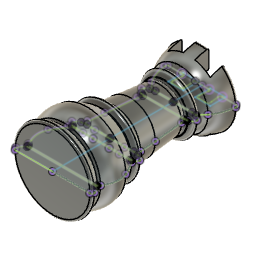
Rook v1 (Autodesk Fusion 360 design; units mm, degrees)
Autodesk Fusion 360 part; units mm, degrees
sketch "Sketch1" plane through (0, 0, 0) normal (0, 0, 1) x (1, 0, 0)
  spline S0 degree 3 poles (56.456539, 22.484084) (57.156363, 22.57219) (57.847984, 22.484877) (58.537222, 22.508691) knots 0 0 0 0 1 1 1 1
  spline S1 degree 3 poles (58.537222, 22.508691) (58.763177, 22.516363) (58.702853, 22.354174) (58.697031, 22.252309) knots 0 0 0 0 1 1 1 1
  spline S2 degree 3 poles (58.697031, 22.252309) (58.67322, 21.863107) (58.623744, 21.475229) (58.598079, 21.086026) knots 0 0 0 0 1 1 1 1
  spline S3 degree 3 poles (58.598079, 21.086026) (58.582996, 20.853723) (58.580618, 20.671953) (58.947593, 20.719578) knots 0 0 0 0 1 1 1 1
  spline S4 degree 3 poles (58.947593, 20.719578) (59.209795, 20.753444) (59.503749, 20.742332) (59.773887, 20.712434) knots 0 0 0 0 1 1 1 1
  spline S5 degree 3 poles (59.773887, 20.712434) (60.200662, 20.665073) (60.237966, 20.861395) (60.18505, 21.195829) knots 0 0 0 0 1 1 1 1
  spline S6 degree 3 poles (60.18505, 21.195829) (60.133454, 21.521267) (60.12102, 21.853318) (60.065988, 22.177961) knots 0 0 0 0 1 1 1 1
  spline S7 degree 3 poles (60.065988, 22.177961) (60.023654, 22.427199) (60.126313, 22.516099) (60.35253, 22.515834) knots 0 0 0 0 1 1 1 1
  spline S8 degree 3 poles (60.35253, 22.515834) (60.976418, 22.515041) (61.600835, 22.513981) (62.224194, 22.510277) knots 0 0 0 0 1 1 1 1
  spline S9 degree 3 poles (62.224194, 22.510277) (62.435595, 22.509219) (62.55651, 22.462917) (62.509149, 22.18775) knots 0 0 0 0 1 1 1 1
  spline S10 degree 3 poles (62.509149, 22.18775) (62.338229, 21.195827) (62.099311, 20.209461) (61.466161, 19.424177) knots 0 0 0 0 1 1 1 1
  spline S11 degree 3 poles (61.466161, 19.424177) (61.153689, 19.037092) (60.831954, 18.580155) (60.102764, 18.618255) knots 0 0 0 0 1 1 1 1
  spline S12 degree 3 poles (60.102764, 18.618255) (58.379266, 18.708212) (56.648097, 18.640746) (54.920106, 18.632805) knots 0 0 0 0 1 1 1 1
  spline S13 degree 3 poles (54.920106, 18.632805) (54.658696, 18.631747) (54.426657, 18.681752) (54.236156, 18.877545) knots 0 0 0 0 1 1 1 1
  spline S14 degree 3 poles (54.236156, 18.877545) (53.326518, 19.815493) (52.892868, 20.96405) (52.749728, 22.23987) knots 0 0 0 0 1 1 1 1
  spline S15 degree 3 poles (52.749728, 22.23987) (52.735707, 22.362372) (52.676703, 22.530647) (52.922234, 22.526414) knots 0 0 0 0 1 1 1 1
  spline S16 degree 3 poles (52.922234, 22.526414) (53.561734, 22.515302) (54.201759, 22.517153) (54.841521, 22.515566) knots 0 0 0 0 1 1 1 1
  spline S17 degree 3 poles (54.841521, 22.515566) (55.083084, 22.514773) (55.194475, 22.428253) (55.153728, 22.158379) knots 0 0 0 0 1 1 1 1
  spline S18 degree 3 poles (55.153728, 22.158379) (55.095786, 21.773674) (55.075939, 21.38315) (55.035724, 20.9958) knots 0 0 0 0 1 1 1 1
  spline S19 degree 3 poles (55.035724, 20.9958) (55.019054, 20.840491) (55.031489, 20.687296) (55.22834, 20.70661) knots 0 0 0 0 1 1 1 1
  spline S20 degree 3 poles (55.22834, 20.70661) (55.642942, 20.747885) (56.060984, 20.639936) (56.475587, 20.749738) knots 0 0 0 0 1 1 1 1
  spline S21 degree 3 poles (56.475587, 20.749738) (56.580627, 20.777784) (56.661323, 20.764026) (56.646244, 20.908487) knots 0 0 0 0 1 1 1 1
  spline S22 degree 3 poles (56.646244, 20.908487) (56.591209, 21.428132) (56.617402, 21.957033) (56.456539, 22.484084) knots 0 0 0 0 1 1 1 1
  line L0 (62.280812, 3.156799) -> (52.878314, 3.156799)
  spline S23 degree 3 poles (52.878314, 3.156799) (52.587008, 3.053612) (52.435136, 2.800139) (52.282472, 2.325741) knots 0 0 0 0 1 1 1 1
  spline S24 degree 3 poles (52.282472, 2.325741) (52.173992, 1.988399) (52.268184, 1.946856) (52.556579, 1.947652) knots 0 0 0 0 1 1 1 1
  spline S25 degree 3 poles (52.556579, 1.947652) (54.118415, 1.953473) (55.68025, 1.953207) (57.241819, 1.952149) knots 0 0 0 0 1 1 1 1
  spline S26 degree 3 poles (57.241819, 1.952149) (59.060034, 1.950825) (60.877458, 1.951354) (62.694882, 1.939185) knots 0 0 0 0 1 1 1 1
  spline S27 degree 3 poles (62.694882, 1.939185) (62.988569, 1.93707) (63.017936, 2.059043) (62.963434, 2.299814) knots 0 0 0 0 1 1 1 1
  spline S28 degree 3 poles (62.963434, 2.299814) (62.85046, 2.797495) (62.650169, 3.059434) (62.280812, 3.156799) knots 0 0 0 0 1 1 1 1
  line L1 (54.363684, 17.329206) -> (60.721888, 17.329206)
  spline S29 degree 3 poles (60.721888, 17.329206) (60.74861, 17.332117) (60.774803, 17.334499) (60.801263, 17.33873) knots 0 0 0 0 1 1 1 1
  spline S30 degree 3 poles (60.801263, 17.33873) (61.148662, 17.392441) (61.432293, 17.710469) (61.383875, 17.990927) knots 0 0 0 0 1 1 1 1
  spline S31 degree 3 poles (61.383875, 17.990927) (61.323284, 18.342823) (61.112412, 18.510303) (60.744375, 18.508717) knots 0 0 0 0 1 1 1 1
  spline S32 degree 3 poles (60.744375, 18.508717) (58.68433, 18.498135) (56.624282, 18.493634) (54.564503, 18.493634) knots 0 0 0 0 1 1 1 1
  spline S33 degree 3 poles (54.564503, 18.493634) (54.29357, 18.493634) (54.06841, 18.427488) (53.955432, 18.169255) knots 0 0 0 0 1 1 1 1
  spline S34 degree 3 poles (53.955432, 18.169255) (53.80012, 17.81419) (54.004379, 17.450121) (54.363684, 17.329206) knots 0 0 0 0 1 1 1 1
  spline S35 degree 3 poles (61.03277, 12.609569) (60.880635, 13.946245) (60.75972, 15.284769) (60.63325, 16.623298) knots 0 0 0 0 1 1 1 1
  spline S36 degree 3 poles (60.63325, 16.623298) (60.597004, 17.008001) (60.577953, 17.137119) (60.39195, 17.178925) knots 0 0 0 0 1 1 1 1
  line L2 (60.39195, 17.178925) -> (54.82882, 17.178925)
  spline S37 degree 3 poles (54.82882, 17.178925) (54.745742, 17.150087) (54.684356, 17.080235) (54.671393, 16.909315) knots 0 0 0 0 1 1 1 1
  spline S38 degree 3 poles (54.671393, 16.909315) (54.606834, 16.020844) (54.513965, 15.134226) (54.427977, 14.247607) knots 0 0 0 0 1 1 1 1
  spline S39 degree 3 poles (54.427977, 14.247607) (54.289601, 12.822561) (54.14699, 11.398044) (54.003584, 9.94072) knots 0 0 0 0 1 1 1 1
  spline S40 degree 3 poles (54.003584, 9.94072) (54.767701, 9.94072) (55.54531, 9.941778) (56.323452, 9.94072) knots 0 0 0 0 1 1 1 1
  spline S41 degree 3 poles (56.323452, 9.94072) (57.814644, 9.939133) (59.30557, 9.945746) (60.796233, 9.927756) knots 0 0 0 0 1 1 1 1
  spline S42 degree 3 poles (60.796233, 9.927756) (61.150774, 9.923259) (61.249992, 10.040734) (61.223537, 10.385222) knots 0 0 0 0 1 1 1 1
  spline S43 degree 3 poles (61.223537, 10.385222) (61.167181, 11.127639) (61.116643, 11.875348) (61.03277, 12.609569) knots 0 0 0 0 1 1 1 1
  line L3 (53.457485, 8.771787) -> (53.993002, 8.771787)
  spline S44 degree 3 poles (53.993002, 8.771787) (53.999087, 8.771787) (54.004908, 8.771787) (54.010992, 8.771787) knots 0 0 0 0 1 1 1 1
  line L4 (54.010992, 8.771787) -> (61.651365, 8.771787)
  spline S45 degree 3 poles (61.651365, 8.771787) (62.032894, 8.81465) (62.241122, 8.99192) (62.229479, 9.265765) knots 0 0 0 0 1 1 1 1
  spline S46 degree 3 poles (62.229479, 9.265765) (62.215191, 9.602845) (61.949284, 9.787257) (61.473566, 9.788848) knots 0 0 0 0 1 1 1 1
  spline S47 degree 3 poles (61.473566, 9.788848) (60.849944, 9.791492) (60.22579, 9.792021) (59.602168, 9.793612) knots 0 0 0 0 1 1 1 1
  spline S48 degree 3 poles (59.602168, 9.793612) (58.091929, 9.796256) (56.581951, 9.800491) (55.071441, 9.80102) knots 0 0 0 0 1 1 1 1
  spline S49 degree 3 poles (55.071441, 9.80102) (54.615562, 9.801815) (54.160216, 9.793612) (53.704341, 9.788319) knots 0 0 0 0 1 1 1 1
  spline S50 degree 3 poles (53.704341, 9.788319) (53.337099, 9.783821) (53.15586, 9.54596) (53.153478, 9.229785) knots 0 0 0 0 1 1 1 1
  spline S51 degree 3 poles (53.153478, 9.229785) (53.151625, 8.997742) (53.253755, 8.832111) (53.457485, 8.771787) knots 0 0 0 0 1 1 1 1
  spline S52 degree 3 poles (62.913429, 6.665177) (62.658635, 7.290651) (62.269169, 7.834901) (61.951403, 8.421744) knots 0 0 0 0 1 1 1 1
  spline S53 degree 3 poles (61.951403, 8.421744) (61.854566, 8.600601) (61.692375, 8.613039) (61.520397, 8.612773) knots 0 0 0 0 1 1 1 1
  spline S54 degree 3 poles (61.520397, 8.612773) (61.033299, 8.612773) (60.545937, 8.612506) (60.058839, 8.612506) knots 0 0 0 0 1 1 1 1
  spline S55 degree 3 poles (60.058839, 8.612506) (59.59476, 8.61224) (59.130944, 8.612506) (58.667132, 8.612506) knots 0 0 0 0 1 1 1 1
  spline S56 degree 3 poles (58.667132, 8.612506) (58.667132, 8.61568) (58.667132, 8.618328) (58.667132, 8.621501) knots 0 0 0 0 1 1 1 1
  line L5 (58.667132, 8.621501) -> (53.760168, 8.621501)
  spline S57 degree 3 poles (53.760168, 8.621501) (53.698786, 8.6088) (53.644017, 8.580225) (53.600625, 8.516727) knots 0 0 0 0 1 1 1 1
  spline S58 degree 3 poles (53.600625, 8.516727) (53.178085, 7.898661) (52.733587, 7.289327) (52.377722, 6.633158) knots 0 0 0 0 1 1 1 1
  spline S59 degree 3 poles (52.377722, 6.633158) (51.942482, 5.830146) (52.09938, 4.976601) (52.392272, 4.166448) knots 0 0 0 0 1 1 1 1
  spline S60 degree 3 poles (52.392272, 4.166448) (52.594679, 3.606324) (52.723002, 3.404713) (53.074369, 3.344651) knots 0 0 0 0 1 1 1 1
  line L6 (53.074369, 3.344651) -> (62.303037, 3.344651)
  spline S61 degree 3 poles (62.303037, 3.344651) (62.392466, 3.378782) (62.473694, 3.443075) (62.538782, 3.560021) knots 0 0 0 0 1 1 1 1
  spline S62 degree 3 poles (62.538782, 3.560021) (63.085939, 4.542951) (63.367188, 5.551546) (62.913429, 6.665177) knots 0 0 0 0 1 1 1 1
  line L7 (57.560832, 22.519067) -> (57.560832, 1.951933)
  constraint perpendicular L0 L7
revolve "Revolve1" add sketch "Sketch1" angle 360 about axis through (57.560832, 22.519067, 0) along (0, -1, 0) contours S0 S1 S2 S3 S4 S5 S6 S7 S8 S9 S10 S11 S12 L7 | L0 S26 S27 S28 L7 | L1 S29 S30 S31 S32 L7 | S35 S36 L2 S41 S42 S43 L7 | L4 S45 S46 S47 S48 L7 | S52 S53 S54 S55 S56 L5 L6 S61 S62 L7 picked at (58.843066, 19.331093) picked at (60.845509, 2.349306) picked at (59.675698, 18.111637) picked at (58.718145, 13.243028) picked at (59.604789, 9.112395) picked at (59.974236, 5.100603) makes body 1 at (58.916375, 8.771787, 0.750935) makes body 2 at (60.984842, 20.949003, 3.177016) makes body 3 at (54.215916, 4.393756, -4.194392) makes body 4 at (60.885542, 13.946793, -0.165929) makes body 5 at (55.173184, 18.504928, 0) makes body 6 at (53.710141, 1.945857, 0)
sketch "Sketch2" plane through (0, 0, 0) normal (0, 0, 1) x (1, 0, 0)
  spline S0 degree 3 poles (58.537222, 22.508691) (58.374743, 22.503077) (58.212157, 22.503642) (57.88746, 22.509584) (57.725237, 22.514953) (57.562009, 22.519037) (57.561421, 22.519052) (57.560832, 22.519067) knots -0.09770796 -0.09770796 -0.09770796 -0.09770796 -0.04880692 -0.04880692 0 0 0.0001766 0.0001766 0.0001766 0.0001766
  spline S1 degree 3 poles (57.560832, 22.519067) (57.560244, 22.519052) (57.559655, 22.519037) (57.396428, 22.514953) (57.234205, 22.509584) (56.909507, 22.503642) (56.746921, 22.503077) (56.584443, 22.508691) knots -0.09762764 -0.09762764 -0.09762764 -0.09762764 -0.0974515 -0.0974515 -0.04877269 -0.04877269 0 0 0 0
  spline S2 degree 3 poles (54.769134, 22.515834) (54.457108, 22.515438) (54.145089, 22.514974) (53.521297, 22.513321) (53.209294, 22.51213) (52.89747, 22.510277) knots -0.18715063 -0.18715063 -0.18715063 -0.18715063 -0.09354867 -0.09354867 0 0 0 0
  spline S3 degree 3 poles (52.89747, 22.510277) (52.827114, 22.509925) (52.766785, 22.504562) (52.69966, 22.480309) (52.680993, 22.470735) (52.648886, 22.44481) (52.636343, 22.429528) (52.615182, 22.390035) (52.607851, 22.364537) (52.599958, 22.295101) (52.602344, 22.246846) (52.612515, 22.18775) knots -0.0820162 -0.0820162 -0.0820162 -0.0820162 -0.0542049 -0.0542049 -0.04266662 -0.04266662 -0.03149039 -0.03149039 -0.01798963 -0.01798963 0 0 0 0
  spline S4 degree 3 poles (52.612515, 22.18775) (52.704342, 21.654838) (52.818349, 21.108717) (53.164161, 20.172799) (53.370971, 19.777077) (53.655503, 19.424177) knots -0.29910345 -0.29910345 -0.29910345 -0.29910345 -0.13599545 -0.13599545 0 0 0 0
  spline S5 degree 3 poles (53.655503, 19.424177) (53.799947, 19.245243) (53.946207, 19.051614) (54.245815, 18.807301) (54.366194, 18.73571) (54.648401, 18.634905) (54.817556, 18.607735) (55.018901, 18.618255) knots -0.21041698 -0.21041698 -0.21041698 -0.21041698 -0.11657514 -0.11657514 -0.06048604 -0.06048604 0 0 0 0
  spline S6 degree 3 poles (55.018901, 18.618255) (55.441953, 18.640336) (55.865388, 18.652927) (56.711898, 18.665556) (57.13505, 18.665613) (57.558935, 18.662608) (57.559884, 18.662601) (57.560832, 18.662594) knots -0.25395917 -0.25395917 -0.25395917 -0.25395917 -0.12688391 -0.12688391 0 0 0.00028462 0.00028462 0.00028462 0.00028462
  spline S7 degree 3 poles (57.560832, 18.662594) (57.561781, 18.662601) (57.56273, 18.662608) (57.986614, 18.665613) (58.409767, 18.665556) (59.256277, 18.652927) (59.679711, 18.640336) (60.102764, 18.618255) knots -0.25427015 -0.25427015 -0.25427015 -0.25427015 -0.2539855 -0.2539855 -0.12708844 -0.12708844 0 0 0 0
  spline S8 degree 3 poles (60.102764, 18.618255) (60.264394, 18.60981) (60.424712, 18.624709) (60.711268, 18.715367) (60.829821, 18.778654) (61.15132, 19.019589) (61.309781, 19.230456) (61.466161, 19.424177) knots -0.16022181 -0.16022181 -0.16022181 -0.16022181 -0.1140258 -0.1140258 -0.07468907 -0.07468907 0 0 0 0
  spline S9 degree 3 poles (61.466161, 19.424177) (61.780203, 19.813677) (61.999008, 20.254625) (62.322223, 21.200122) (62.424919, 21.698927) (62.509149, 22.18775) knots -0.29831003 -0.29831003 -0.29831003 -0.29831003 -0.14880799 -0.14880799 0 0 0 0
  spline S10 degree 3 poles (62.509149, 22.18775) (62.521923, 22.261968) (62.522459, 22.319552) (62.507484, 22.384982) (62.499873, 22.405049) (62.477163, 22.439951) (62.463302, 22.453882) (62.425936, 22.479352) (62.401518, 22.489107) (62.331844, 22.506403) (62.281346, 22.509991) (62.224194, 22.510277) knots -0.06670843 -0.06670843 -0.06670843 -0.06670843 -0.04653663 -0.04653663 -0.03707383 -0.03707383 -0.0281827 -0.0281827 -0.0171458 -0.0171458 0 0 0 0
  spline S11 degree 3 poles (62.224194, 22.510277) (61.912371, 22.51213) (61.600368, 22.513321) (60.976576, 22.514974) (60.664556, 22.515438) (60.35253, 22.515834) knots -0.1871624 -0.1871624 -0.1871624 -0.1871624 -0.09360785 -0.09360785 0 0 0 0
  spline S12 degree 3 poles (61.383875, 17.990927) (61.371233, 18.064349) (61.350691, 18.137626) (61.289893, 18.262797) (61.253212, 18.315101) (61.156565, 18.405554) (61.099173, 18.439486) (60.943653, 18.497621) (60.84244, 18.509139) (60.744375, 18.508717) knots -0.09136626 -0.09136626 -0.09136626 -0.09136626 -0.06904077 -0.06904077 -0.04970491 -0.04970491 -0.02941973 -0.02941973 0 0 0 0
  spline S13 degree 3 poles (60.744375, 18.508717) (60.213782, 18.505991) (59.683186, 18.503669) (58.623067, 18.499782) (58.093541, 18.498215) (57.562954, 18.496993) (57.561893, 18.496991) (57.560832, 18.496988) knots -0.31803786 -0.31803786 -0.31803786 -0.31803786 -0.15885803 -0.15885803 0 0 0.00031833 0.00031833 0.00031833 0.00031833
  spline S14 degree 3 poles (57.560832, 18.496988) (57.559771, 18.496991) (57.55871, 18.496993) (57.028124, 18.498215) (56.498597, 18.499782) (55.438478, 18.503669) (54.907882, 18.505991) (54.37729, 18.508717) knots -0.31835618 -0.31835618 -0.31835618 -0.31835618 -0.31803785 -0.31803785 -0.15917983 -0.15917983 0 0 0 0
  spline S15 degree 3 poles (54.37729, 18.508717) (54.296104, 18.509067) (54.212949, 18.501231) (54.071543, 18.461297) (54.012165, 18.434335) (53.905773, 18.356177) (53.862601, 18.307465) (53.780977, 18.171779) (53.753377, 18.081456) (53.73779, 17.990927) knots -0.09144385 -0.09144385 -0.09144385 -0.09144385 -0.06709321 -0.06709321 -0.0474261 -0.0474261 -0.02755825 -0.02755825 0 0 0 0
  spline S16 degree 3 poles (53.73779, 17.990927) (53.732259, 17.958893) (53.731074, 17.926446) (53.736525, 17.861051) (53.743271, 17.82851) (53.774297, 17.730212) (53.809658, 17.667786) (53.911026, 17.539107) (53.986746, 17.474153) (54.149967, 17.382164) (54.233748, 17.352127) (54.320401, 17.33873) knots -0.09982241 -0.09982241 -0.09982241 -0.09982241 -0.08937801 -0.08937801 -0.07873973 -0.07873973 -0.05627132 -0.05627132 -0.02630483 -0.02630483 0 0 0 0
  spline S17 degree 3 poles (54.320401, 17.33873) (54.333582, 17.336622) (54.346705, 17.334971) (54.373201, 17.331983) (54.386413, 17.330662) (54.399777, 17.329206) knots -0.00808903 -0.00808903 -0.00808903 -0.00808903 -0.004033 -0.004033 0 0 0 0
  line L0 (54.399777, 17.329206) -> (60.721888, 17.329206)
  spline S18 degree 3 poles (60.721888, 17.329206) (60.735252, 17.330662) (60.748464, 17.331983) (60.77496, 17.334971) (60.788082, 17.336622) (60.801263, 17.33873) knots -0.00798643 -0.00798643 -0.00798643 -0.00798643 -0.00400459 -0.00400459 0 0 0 0
  spline S19 degree 3 poles (60.801263, 17.33873) (60.867003, 17.348894) (60.931067, 17.368623) (61.050516, 17.423412) (61.106285, 17.458209) (61.220098, 17.551016) (61.276094, 17.613736) (61.347767, 17.735279) (61.370588, 17.791164) (61.390716, 17.896283) (61.391987, 17.94394) (61.383875, 17.990927) knots -0.09567143 -0.09567143 -0.09567143 -0.09567143 -0.07587052 -0.07587052 -0.05653582 -0.05653582 -0.03209894 -0.03209894 -0.0143047 -0.0143047 0 0 0 0
  spline S20 degree 3 poles (60.63325, 16.623298) (60.617073, 16.794999) (60.604341, 16.915787) (60.567993, 17.035681) (60.55522, 17.064461) (60.524331, 17.110037) (60.506489, 17.127955) (60.459215, 17.158882) (60.428905, 17.170619) (60.39195, 17.178925) knots -0.05853717 -0.05853717 -0.05853717 -0.05853717 -0.03217875 -0.03217875 -0.02133432 -0.02133432 -0.01136314 -0.01136314 0 0 0 0
  line L1 (60.39195, 17.178925) -> (54.729715, 17.178925)
  spline S21 degree 3 poles (54.729715, 17.178925) (54.701957, 17.172686) (54.67735, 17.164396) (54.634852, 17.142331) (54.616674, 17.128789) (54.581142, 17.089941) (54.565606, 17.0631) (54.520361, 16.944103) (54.506538, 16.815653) (54.488414, 16.623298) knots -0.1176784 -0.1176784 -0.1176784 -0.1176784 -0.09869434 -0.09869434 -0.080581 -0.080581 -0.05796194 -0.05796194 0 0 0 0
  spline S22 degree 3 poles (54.488414, 16.623298) (54.425179, 15.954027) (54.363334, 15.284781) (54.233192, 13.946373) (54.16494, 13.277712) (54.088895, 12.609569) knots -0.40337656 -0.40337656 -0.40337656 -0.40337656 -0.20173702 -0.20173702 0 0 0 0
  spline S23 degree 3 poles (54.088895, 12.609569) (54.046805, 12.24112) (54.013165, 11.869636) (53.953036, 11.129044) (53.926302, 10.756379) (53.898128, 10.385222) knots -0.22265566 -0.22265566 -0.22265566 -0.22265566 -0.11166739 -0.11166739 0 0 0 0
  spline S24 degree 3 poles (53.898128, 10.385222) (53.891162, 10.294514) (53.892889, 10.219765) (53.912654, 10.12536) (53.923602, 10.092737) (53.956583, 10.03705) (53.976475, 10.014898) (54.029385, 9.975775) (54.063852, 9.960036) (54.164225, 9.933102) (54.236732, 9.926631) (54.325432, 9.927756) knots -0.11352103 -0.11352103 -0.11352103 -0.11352103 -0.07998527 -0.07998527 -0.06178687 -0.06178687 -0.04538733 -0.04538733 -0.02661194 -0.02661194 0 0 0 0
  spline S25 degree 3 poles (54.325432, 9.927756) (54.86461, 9.934263) (55.403816, 9.937551) (56.481216, 9.940792) (57.019568, 9.94075) (57.558693, 9.940592) (57.559763, 9.940591) (57.560832, 9.940591) knots -0.32314047 -0.32314047 -0.32314047 -0.32314047 -0.16141641 -0.16141641 0 0 0.00032094 0.00032094 0.00032094 0.00032094
  spline S26 degree 3 poles (57.560832, 9.940591) (57.561902, 9.940591) (57.562972, 9.940592) (58.102096, 9.94075) (58.640449, 9.940792) (59.717849, 9.937551) (60.257054, 9.934263) (60.796233, 9.927756) knots -0.32354397 -0.32354397 -0.32354397 -0.32354397 -0.32322295 -0.32322295 -0.16176534 -0.16176534 0 0 0 0
  spline S27 degree 3 poles (60.796233, 9.927756) (60.889885, 9.926568) (60.965718, 9.933891) (61.05835, 9.961136) (61.089564, 9.97458) (61.141787, 10.011742) (61.16201, 10.033244) (61.196822, 10.089261) (61.209828, 10.125267) (61.228922, 10.227231) (61.230157, 10.299022) (61.223537, 10.385222) knots -0.11088292 -0.11088292 -0.11088292 -0.11088292 -0.07792587 -0.07792587 -0.06034536 -0.06034536 -0.04448261 -0.04448261 -0.02593617 -0.02593617 0 0 0 0
  spline S28 degree 3 poles (61.223537, 10.385222) (61.195363, 10.756379) (61.168629, 11.129044) (61.108499, 11.869636) (61.074859, 12.24112) (61.03277, 12.609569) knots -0.22318833 -0.22318833 -0.22318833 -0.22318833 -0.1112538 -0.1112538 0 0 0 0
  spline S29 degree 3 poles (61.03277, 12.609569) (60.956725, 13.277712) (60.888473, 13.946373) (60.758331, 15.284781) (60.696486, 15.954027) (60.63325, 16.623298) knots -0.40344878 -0.40344878 -0.40344878 -0.40344878 -0.20167565 -0.20167565 0 0 0 0
  spline S30 degree 3 poles (61.473566, 9.788848) (61.161704, 9.79017) (60.849682, 9.790963) (60.225912, 9.792286) (59.914, 9.792816) (59.602168, 9.793612) knots -0.18705796 -0.18705796 -0.18705796 -0.18705796 -0.09354994 -0.09354994 0 0 0 0
  spline S31 degree 3 poles (59.602168, 9.793612) (59.261938, 9.794207) (58.921724, 9.794884) (58.242118, 9.796275) (57.902752, 9.79699) (57.562532, 9.797667) (57.561682, 9.797669) (57.560832, 9.79767) knots -0.20388271 -0.20388271 -0.20388271 -0.20388271 -0.10181134 -0.10181134 0 0 0.00025491 0.00025491 0.00025491 0.00025491
  spline S32 degree 3 poles (57.560832, 9.79767) (57.559983, 9.797669) (57.559133, 9.797667) (57.218913, 9.79699) (56.879547, 9.796275) (56.19994, 9.794884) (55.859727, 9.794207) (55.519496, 9.793612) knots -0.20413342 -0.20413342 -0.20413342 -0.20413342 -0.20387852 -0.20387852 -0.10206927 -0.10206927 0 0 0 0
  spline S33 degree 3 poles (55.519496, 9.793612) (55.207664, 9.792816) (54.895752, 9.792286) (54.271983, 9.790963) (53.959961, 9.79017) (53.648099, 9.788848) knots -0.18716087 -0.18716087 -0.18716087 -0.18716087 -0.09355947 -0.09355947 0 0 0 0
  spline S34 degree 3 poles (53.648099, 9.788848) (53.514196, 9.7884) (53.349868, 9.773361) (53.146946, 9.687569) (53.089981, 9.653496) (52.997878, 9.568248) (52.963243, 9.521042) (52.909068, 9.403756) (52.89514, 9.33546) (52.892186, 9.265765) knots -0.10487728 -0.10487728 -0.10487728 -0.10487728 -0.05859661 -0.05859661 -0.03878048 -0.03878048 -0.02092724 -0.02092724 0 0 0 0
  spline S35 degree 3 poles (52.892186, 9.265765) (52.88987, 9.211311) (52.896108, 9.157352) (52.93035, 9.057022) (52.956198, 9.01327) (53.03364, 8.925834) (53.087713, 8.888083) (53.232322, 8.816348) (53.339888, 8.786438) (53.4703, 8.771787) knots -0.10961904 -0.10961904 -0.10961904 -0.10961904 -0.08727673 -0.08727673 -0.06613161 -0.06613161 -0.03936965 -0.03936965 0 0 0 0
  line L2 (53.4703, 8.771787) -> (61.651365, 8.771787)
  spline S36 degree 3 poles (61.651365, 8.771787) (61.787758, 8.78711) (61.901901, 8.819568) (62.042742, 8.89461) (62.089669, 8.928669) (62.162031, 9.008605) (62.187998, 9.050879) (62.224887, 9.151893) (62.231913, 9.208507) (62.229479, 9.265765) knots -0.08015416 -0.08015416 -0.08015416 -0.08015416 -0.0495612 -0.0495612 -0.03228718 -0.03228718 -0.01719302 -0.01719302 0 0 0 0
  spline S37 degree 3 poles (62.229479, 9.265765) (62.227906, 9.30288) (62.223211, 9.33982) (62.206605, 9.409751) (62.195269, 9.44248) (62.153974, 9.528169) (62.117821, 9.575356) (62.014936, 9.66664) (61.945981, 9.703195) (61.74812, 9.773579) (61.606594, 9.788403) (61.473566, 9.788848) knots -0.10288603 -0.10288603 -0.10288603 -0.10288603 -0.0917153 -0.0917153 -0.08127082 -0.08127082 -0.06310779 -0.06310779 -0.03990875 -0.03990875 0 0 0 0
  line L3 (58.667132, 8.612506) -> (58.667132, 8.621501)
  line L4 (58.667132, 8.621501) -> (56.454533, 8.621501)
  line L5 (56.454533, 8.621501) -> (56.454533, 8.612506)
  spline S38 degree 3 poles (56.454533, 8.612506) (56.222621, 8.612506) (55.990723, 8.61244) (55.526742, 8.612373) (55.294827, 8.612373) (55.062826, 8.612506) knots -0.13917207 -0.13917207 -0.13917207 -0.13917207 -0.06960016 -0.06960016 0 0 0 0
  spline S39 degree 3 poles (55.062826, 8.612506) (54.819277, 8.612506) (54.575662, 8.612573) (54.088432, 8.612706) (53.844817, 8.612773) (53.601267, 8.612773) knots -0.14612965 -0.14612965 -0.14612965 -0.14612965 -0.07306482 -0.07306482 0 0 0 0
  spline S40 degree 3 poles (53.601267, 8.612773) (53.516407, 8.612904) (53.433231, 8.610003) (53.322111, 8.572442) (53.288314, 8.554684) (53.22116, 8.500326) (53.192707, 8.463201) (53.170261, 8.421744) knots -0.04919678 -0.04919678 -0.04919678 -0.04919678 -0.02584318 -0.02584318 -0.01414297 -0.01414297 0 0 0 0
  spline S41 degree 3 poles (53.170261, 8.421744) (53.01139, 8.128343) (52.834563, 7.845537) (52.494571, 7.266725) (52.335019, 6.976407) (52.208236, 6.665177) knots -0.20038004 -0.20038004 -0.20038004 -0.20038004 -0.10081886 -0.10081886 0 0 0 0
  spline S42 degree 3 poles (52.208236, 6.665177) (52.101159, 6.402385) (52.029004, 6.1307) (51.969911, 5.585617) (51.978586, 5.324684) (52.102462, 4.54774) (52.310276, 4.049739) (52.582882, 3.560021) knots -0.34467335 -0.34467335 -0.34467335 -0.34467335 -0.25325087 -0.25325087 -0.16814395 -0.16814395 0 0 0 0
  spline S43 degree 3 poles (52.582882, 3.560021) (52.611668, 3.5083) (52.647148, 3.460524) (52.729401, 3.387953) (52.771494, 3.36264) (52.818628, 3.344651) knots -0.03295648 -0.03295648 -0.03295648 -0.03295648 -0.0151349 -0.0151349 0 0 0 0
  line L6 (52.818628, 3.344651) -> (62.303037, 3.344651)
  spline S44 degree 3 poles (62.303037, 3.344651) (62.350171, 3.36264) (62.392263, 3.387953) (62.474517, 3.460524) (62.509996, 3.5083) (62.538782, 3.560021) knots -0.03283825 -0.03283825 -0.03283825 -0.03283825 -0.01775765 -0.01775765 0 0 0 0
  spline S45 degree 3 poles (62.538782, 3.560021) (62.708796, 3.865438) (62.860864, 4.187216) (63.073892, 4.843347) (63.136576, 5.173485) (63.143512, 5.913031) (63.064162, 6.295241) (62.913429, 6.665177) knots -0.32649986 -0.32649986 -0.32649986 -0.32649986 -0.22151625 -0.22151625 -0.11983982 -0.11983982 0 0 0 0
  spline S46 degree 3 poles (62.913429, 6.665177) (62.786646, 6.976407) (62.627094, 7.266725) (62.287101, 7.845537) (62.110275, 8.128343) (61.951403, 8.421744) knots -0.20145625 -0.20145625 -0.20145625 -0.20145625 -0.10009591 -0.10009591 0 0 0 0
  spline S47 degree 3 poles (61.951403, 8.421744) (61.92973, 8.461773) (61.902422, 8.49783) (61.836561, 8.55283) (61.802111, 8.571384) (61.68964, 8.609962) (61.605872, 8.612905) (61.520397, 8.612773) knots -0.0536314 -0.0536314 -0.0536314 -0.0536314 -0.03874388 -0.03874388 -0.02564237 -0.02564237 0 0 0 0
  spline S48 degree 3 poles (61.520397, 8.612773) (61.276848, 8.612773) (61.033233, 8.612706) (60.546003, 8.612573) (60.302388, 8.612506) (60.058839, 8.612506) knots -0.14612965 -0.14612965 -0.14612965 -0.14612965 -0.07306482 -0.07306482 0 0 0 0
  spline S49 degree 3 poles (60.058839, 8.612506) (59.826838, 8.612373) (59.594923, 8.612373) (59.130942, 8.61244) (58.899043, 8.612506) (58.667132, 8.612506) knots -0.13917517 -0.13917517 -0.13917517 -0.13917517 -0.06957346 -0.06957346 0 0 0 0
  spline S50 degree 3 poles (62.963434, 2.299814) (62.917283, 2.50312) (62.85677, 2.66646) (62.723, 2.881128) (62.658364, 2.955847) (62.488897, 3.084147) (62.388567, 3.128394) (62.280812, 3.156799) knots -0.10923906 -0.10923906 -0.10923906 -0.10923906 -0.06359449 -0.06359449 -0.03343065 -0.03343065 0 0 0 0
  line L7 (62.280812, 3.156799) -> (52.840852, 3.156799)
  spline S51 degree 3 poles (52.840852, 3.156799) (52.744276, 3.131341) (52.653149, 3.093021) (52.489906, 2.980561) (52.423611, 2.911402) (52.276174, 2.696262) (52.208641, 2.521885) (52.158231, 2.299814) knots -0.15140038 -0.15140038 -0.15140038 -0.15140038 -0.10944904 -0.10944904 -0.0683162 -0.0683162 0 0 0 0
  spline S52 degree 3 poles (52.158231, 2.299814) (52.139263, 2.216019) (52.130462, 2.146668) (52.142618, 2.072145) (52.148368, 2.052927) (52.167076, 2.018499) (52.179095, 2.004243) (52.211735, 1.978019) (52.234023, 1.96659) (52.303713, 1.945018) (52.357906, 1.938689) (52.426783, 1.939185) knots -0.09104391 -0.09104391 -0.09104391 -0.09104391 -0.0577515 -0.0577515 -0.04574884 -0.04574884 -0.03428601 -0.03428601 -0.02066375 -0.02066375 0 0 0 0
  spline S53 degree 3 poles (52.426783, 1.939185) (53.282376, 1.944914) (54.137957, 1.947828) (55.847929, 1.951063) (56.702073, 1.951387) (57.558137, 1.951931) (57.559485, 1.951932) (57.560832, 1.951933) knots -0.51320006 -0.51320006 -0.51320006 -0.51320006 -0.25641481 -0.25641481 0 0 0.00040431 0.00040431 0.00040431 0.00040431
  spline S54 degree 3 poles (57.560832, 1.951933) (57.56218, 1.951932) (57.563528, 1.951931) (58.419591, 1.951387) (59.273736, 1.951063) (60.983708, 1.947828) (61.839289, 1.944914) (62.694882, 1.939185) knots -0.51340094 -0.51340094 -0.51340094 -0.51340094 -0.5129968 -0.5129968 -0.25668354 -0.25668354 0 0 0 0
  spline S55 degree 3 poles (62.694882, 1.939185) (62.733507, 1.938907) (62.774972, 1.940722) (62.844928, 1.952481) (62.873663, 1.960789) (62.915495, 1.982208) (62.931191, 1.993457) (62.957456, 2.022393) (62.966986, 2.039002) (62.982233, 2.081738) (62.985763, 2.109064) (62.985794, 2.184659) (62.977353, 2.238325) (62.963434, 2.299814) knots -0.07854228 -0.07854228 -0.07854228 -0.07854228 -0.0627364 -0.0627364 -0.04966448 -0.04966448 -0.04042979 -0.04042979 -0.03114001 -0.03114001 -0.0189136 -0.0189136 0 0 0 0
  line L8 (52.818628, 3.344651) -> (52.840852, 3.156799)
  line L9 (62.280812, 3.156799) -> (62.303037, 3.344651)
  line L10 (53.4703, 8.771787) -> (53.601267, 8.612773)
  line L11 (61.520397, 8.612773) -> (61.651365, 8.771787)
  line L12 (53.648099, 9.788848) -> (54.325432, 9.927756)
  line L13 (61.473566, 9.788848) -> (60.796233, 9.927756)
  line L14 (54.729715, 17.178925) -> (54.399777, 17.329206)
  line L15 (60.39195, 17.178925) -> (60.721888, 17.329206)
  line L16 (54.37729, 18.508717) -> (55.018901, 18.618255)
  line L17 (60.744375, 18.508717) -> (60.102764, 18.618255)
  line L18 (57.560832, 3.156799) -> (57.560832, 3.344651)
  line L19 (57.560832, 8.771787) -> (57.560832, 8.621501)
  line L20 (57.560832, 9.940591) -> (57.560832, 9.79767)
  line L21 (57.560832, 17.329206) -> (57.560832, 17.178925)
  line L22 (57.560832, 18.662594) -> (57.560832, 18.496988)
  line L23 (56.584443, 22.599999) -> (56.584443, 22.508691)
  line L24 (56.584443, 22.508691) -> (54.799999, 22.508691)
  line L25 (54.799999, 22.508691) -> (54.799999, 22.599999)
  line L26 (54.799999, 22.699999) -> (56.899999, 22.699999)
  line L27 (56.899999, 22.699999) -> (56.899999, 20.6)
  line L28 (56.899999, 20.6) -> (54.799999, 20.6)
  line L29 (54.799999, 20.6) -> (54.799999, 22.699999)
  line L30 (58.499999, 22.699999) -> (60.599999, 22.699999)
  line L31 (60.599999, 22.699999) -> (60.599999, 20.6)
  line L32 (60.599999, 20.6) -> (58.499999, 20.6)
  line L33 (58.499999, 20.6) -> (58.499999, 22.699999)
  dimension "d7" = 2.1
  constraint vertical L23
  constraint horizontal L24
  constraint vertical L25
  constraint horizontal L26
  constraint vertical L27
  constraint horizontal L28
  constraint vertical L29
  constraint horizontal L30
  constraint vertical L31
  constraint horizontal L32
  constraint vertical L33
revolve "Revolve2" add sketch "Sketch2" angle 360 about axis through (57.560832, 22.519067, 0) along (0, -1, 0) contours S7 S13 L17 L22 | L0 L1 L15 L21 | S26 S30 S31 L13 L20 | L2 L3 L4 S48 S49 L11 L19 | L6 L7 L9 L18 picked at (58.408143, 18.592612) picked at (59.558223, 17.279112) picked at (59.319745, 9.88732) picked at (59.29311, 8.721692) picked at (60.714894, 3.282034) bodies 3 1 2 4 5 6
extrude "Extrude1" cut sketch "Sketch2" along normal mid plane 13 contours S1 L24 L27 L28 L29 | S1 L24 L25 L26 L27 L29 | L30 L31 L32 L33 picked at (56.094813, 21.23623) picked at (56.094813, 22.63623) picked at (59.899999, 21.874337) bodies 3
